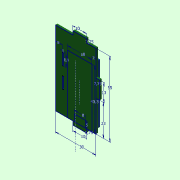
# Autodesk Inventor part: Motherboard_dummy
Saved by Autodesk Inventor 2015 (Build 190159000, 159)
## iProperties
Created: 2014-12-25
Part Number: Motherboard_dummy
Material: ABS Plastic
Document SubType Name: Modeling
Designer: Openlab
Density: 1.06 g/cm^3
Appearance: Smooth - Dark Forest Green
Mass: 9.08054 g
Surface Area: 59.127 cm^2
Volume: 8.56654 cm^3
Author: Openlab
Autodesk Inventor part; units mm, degrees
ref_plane "YZ Plane" through (0, 0, 0) normal (1, 0, 0) x (0, 1, 0)
ref_plane "XZ Plane" through (0, 0, 0) normal (0, 1, 0) x (-1, 0, 0)
ref_plane "XY Plane" through (0, 0, 0) normal (0, 0, 1) x (1, 0, 0)
sketch "Sketch1" plane through (0, 0, 0) normal (0, 1, 0) x (-1, 0, 0)
  line L0 (30, 0) -> (0, 0)
  line L1 (3, 0) -> (3, 43.3)
  line L2 (3, 43.3) -> (21, 43.3)
  line L3 (21, 43.3) -> (21, 0)
  line L4 (15, -19.2684) -> (15, 39.5149) construction
  line L5 (8, 5) -> (16, 5)
  line L6 (16, 5) -> (16, 0)
  line L7 (8, 0) -> (8, 5)
  line L8 (7, 55) -> (7, 57.75)
  line L9 (7, 57.75) -> (17, 57.75)
  line L10 (17, 57.75) -> (17, 55)
  line L11 (0, 55) -> (7, 55)
  line L12 (17, 55) -> (30, 55)
  line L13 (0, 0) -> (0, 55)
  line L14 (30, 55) -> (30, 0)
  line L15 (7, 0) -> (7, -2.75)
  line L16 (7, -2.75) -> (17, -2.75)
  line L17 (17, -2.75) -> (17, 0)
  line L18 (0, 36) -> (-2.75, 36)
  line L19 (-2.75, 36) -> (-2.75, 23)
  line L20 (-2.75, 23) -> (0, 23)
  line L21 (25, 16.4874) -> (25, 24.9874)
  line L22 (25, 24.9874) -> (24, 24.9874)
  line L23 (24, 24.9874) -> (24, 16.4874)
  line L24 (24, 16.4874) -> (25, 16.4874)
  line L25 (24, 31.5442) -> (25, 31.5442)
  line L26 (25, 31.5442) -> (25, 40.0442)
  line L27 (25, 40.0442) -> (24, 40.0442)
  line L28 (24, 40.0442) -> (24, 31.5442)
  line L29 (12, 13) -> (12, 28.6373) construction
  point P0 (0, 0)
  point P1 (0, 0)
  point P2 (0, 0)
  point P3 (0, 0)
  dimension "d47" = 18
  dimension "d49" = 43.3
  dimension "d50" = 5
  dimension "d51" = 8
  dimension "d52" = 30
  dimension "d53" = 55
  dimension "d123" = 10
  dimension "d126" = 2.75
  dimension "d134" = 10
  dimension "d136" = 2.75
  dimension "d146" = 2.75
  dimension "d147" = 13
  dimension "d149" = 23
  dimension "d151" = 8.5
  dimension "d153" = 1
  dimension "d155" = 5
  dimension "d156" = 3
  constraints: 60 end point, 19 perpendicular, 8 point on line, 4 coincident, 4 vertical, 2 collinear, 2 equal length, 2 parallel, 1 horizontal, 1 horizontal alignment, 5 other
  measures "d47" distance of L2.start L2.end
  measures "d49" distance of L1.start L2.start
  measures "d50" distance of L7.start L5.start
  measures "d51" distance of L5.start L5.end
  measures "d52" distance of L0.end L0.start
  measures "d53" distance of L0.end L11.start
  measures "d123" distance of L8.end L9.end
  measures "d126" distance of L8.start L8.end
  measures "d134" distance of L15.end L16.end
  measures "d136" distance of L15.start L15.end
  measures "d146" distance of L18.start L18.end
  measures "d147" distance of L18.end L19.end
  measures "d149" distance between parallel lines of L0 L20
  measures "d151" distance of L27.end L25.start
  measures "d153" distance of L26.end L27.end
  measures "d155" distance between parallel lines of L14 L26
  measures "d156" distance between parallel lines of L1 L13
extrude "Extrusion1" add sketch "Sketch1" along normal blind 1.5
extrude "Extrusion2" add sketch "Sketch1" along normal blind 6 contours L0 L6 L5 L7 L1 L2 L3 | L0 L7 L5 L6
sketch "Sketch2" plane through (0, 0, 0) normal (0, 0, -1) x (-1, 0, 0)
  line L0 (8, 10) -> (16, 10)
  line L1 (16, 10) -> (16, 6)
  line L2 (16, 6) -> (8, 6)
  line L3 (8, 6) -> (8, 10)
  line L4 (0, 0) -> (7, 0) projected
  line L5 (16, 6) -> (16, 10)
  line L6 (12, 9) -> (12, -2.5232) construction
  line L7 (3, 1.5) -> (3, 6) projected
  line L8 (7, 1.5) -> (17, 1.5) projected
  point P0 (30, 0)
  point P1 (21.75, 6)
  point P2 (12, 1.5)
  dimension "d100" = 4
  dimension "d101" = 8
  constraints: 10 end point, 2 parallel, 2 vertical, 1 horizontal, 1 midpoint, 1 perpendicular, 1 point on line, 4 other
  measures "d100" distance of L2.end L0.start
  measures "d101" distance of L0.start L0.end
extrude "Extrusion7" add sketch "Sketch2" along normal blind 1.5
extrude "Extrusion9" cut sketch "Sketch1" along normal blind 10 contours L0 L7 L5 L6
extrude "Extrusion10" add sketch "Sketch1" along normal blind 10 contours L0 L7 L5 L6
body "Solid1"
